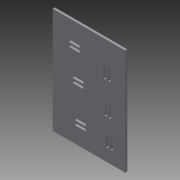
# Autodesk Inventor part: Bottom
Saved by Autodesk Inventor 2015 (Build 190159000, 159)
## iProperties
Created: 2014-09-15
Part Number: Bottom
Material: Generic
Document SubType Name: Modeling
Designer: ehagerup
Density: 1 g/cm^3
Appearance: Default
Author: ehagerup
Autodesk Inventor part; units mm, degrees
ref_plane "YZ Plane" through (0, 0, 0) normal (1, 0, 0) x (0, 1, 0)
ref_plane "XZ Plane" through (0, 0, 0) normal (0, 1, 0) x (-1, 0, 0)
ref_plane "XY Plane" through (0, 0, 0) normal (0, 0, 1) x (1, 0, 0)
sketch "Sketch1" plane through (0, 0, 0) normal (0, 1, 0) x (-1, 0, 0)
  line L0 (52.9273, -103.1635) -> (52.4273, -103.1635)
  line L1 (49.4273, -103.1635) -> (50.9273, -103.1635)
  line L2 (47.9273, -103.1635) -> (47.4273, -103.1635)
  line L3 (58.4273, -103.1635) -> (59.9273, -103.1635)
  line L4 (52.9273, -109.1635) -> (52.4273, -109.1635)
  line L5 (49.4273, -109.1635) -> (50.9273, -109.1635)
  line L6 (50.9273, -106.1635) -> (49.4273, -106.1635)
  line L7 (47.4273, -106.1635) -> (47.9273, -106.1635)
  line L8 (47.9273, -109.1635) -> (47.4273, -109.1635)
  line L9 (52.4273, -106.1635) -> (52.9273, -106.1635)
  line L10 (58.4273, -109.1635) -> (59.9273, -109.1635)
  line L11 (59.9273, -106.1635) -> (58.4273, -106.1635)
  line L12 (50.9273, -112.1635) -> (49.4273, -112.1635)
  line L13 (47.4273, -112.1635) -> (47.9273, -112.1635)
  line L14 (52.4273, -112.1635) -> (52.9273, -112.1635)
  line L15 (59.9273, -112.1635) -> (58.4273, -112.1635)
  line L16 (15.9643, -33.5509) -> (15.9643, -36.0509)
  line L17 (18.9643, -33.5509) -> (18.9643, -36.0509)
  line L18 (14.8002, -77.3245) -> (14.8002, -79.8245)
  line L19 (17.8002, -77.3245) -> (17.8002, -79.8245)
  line L20 (15.7165, -102.0792) -> (15.7165, -104.5792)
  line L21 (12.7165, -114.0792) -> (12.7165, -116.5792)
  line L22 (15.7165, -114.0792) -> (15.7165, -116.5792)
  line L23 (-7.557, 11.8403) -> (92.5214, 11.8403)
  line L24 (92.5214, 11.8403) -> (92.5214, -134.0855)
  line L25 (92.5214, -134.0855) -> (-7.557, -134.0855)
  line L26 (-7.557, -134.0855) -> (-7.557, 11.8403)
  line L27 (17.8002, -65.0745) -> (20.8002, -65.0745)
  line L28 (20.8002, -65.0745) -> (20.8002, -80.0745)
  line L29 (20.8002, -80.0745) -> (17.8002, -80.0745)
  line L30 (17.8002, -80.0745) -> (17.8002, -65.0745)
  line L31 (14.8002, -65.0745) -> (11.8002, -65.0745)
  line L32 (11.8002, -65.0745) -> (11.8002, -80.0745)
  line L33 (11.8002, -80.0745) -> (14.8002, -80.0745)
  line L34 (14.8002, -80.0745) -> (14.8002, -65.0745)
  line L35 (12.7165, -101.8292) -> (9.7165, -101.8292)
  line L36 (9.7165, -101.8292) -> (9.7165, -116.8292)
  line L37 (9.7165, -116.8292) -> (12.7165, -116.8292)
  line L38 (12.7165, -116.8292) -> (12.7165, -101.8292)
  line L39 (15.7165, -101.8292) -> (18.7165, -101.8292)
  line L40 (18.7165, -101.8292) -> (18.7165, -116.8292)
  line L41 (18.7165, -116.8292) -> (15.7165, -116.8292)
  line L42 (15.7165, -116.8292) -> (15.7165, -101.8292)
  line L43 (18.9643, -21.3009) -> (21.9643, -21.3009)
  line L44 (21.9643, -21.3009) -> (21.9643, -36.3009)
  line L45 (21.9643, -36.3009) -> (18.9643, -36.3009)
  line L46 (18.9643, -36.3009) -> (18.9643, -21.3009)
  line L47 (15.9643, -21.3009) -> (12.9643, -21.3009)
  line L48 (12.9643, -21.3009) -> (12.9643, -36.3009)
  line L49 (12.9643, -36.3009) -> (15.9643, -36.3009)
  line L50 (15.9643, -36.3009) -> (15.9643, -21.3009)
  line L51 (70.4221, -13.6009) -> (55.4221, -13.6009)
  line L52 (55.4221, -13.6009) -> (55.4221, -16.6009)
  line L53 (55.4221, -16.6009) -> (70.4221, -16.6009)
  line L54 (70.4221, -16.6009) -> (70.4221, -13.6009)
  line L55 (55.4221, -19.6009) -> (70.4221, -19.6009)
  line L56 (70.4221, -19.6009) -> (70.4221, -22.6009)
  line L57 (70.4221, -22.6009) -> (55.4221, -22.6009)
  line L58 (55.4221, -22.6009) -> (55.4221, -19.6009)
  line L59 (65.3229, -54.1341) -> (50.3229, -54.1341)
  line L60 (50.3229, -54.1341) -> (50.3229, -57.1341)
  line L61 (50.3229, -57.1341) -> (65.3229, -57.1341)
  line L62 (65.3229, -57.1341) -> (65.3229, -54.1341)
  line L63 (50.3229, -60.1341) -> (65.3229, -60.1341)
  line L64 (65.3229, -60.1341) -> (65.3229, -63.1341)
  line L65 (65.3229, -63.1341) -> (50.3229, -63.1341)
  line L66 (50.3229, -63.1341) -> (50.3229, -60.1341)
  line L67 (47.1773, -103.1635) -> (62.1773, -103.1635)
  line L68 (62.1773, -103.1635) -> (62.1773, -106.1635)
  line L69 (62.1773, -106.1635) -> (47.1773, -106.1635)
  line L70 (47.1773, -106.1635) -> (47.1773, -103.1635)
  line L71 (62.1773, -109.1635) -> (47.1773, -109.1635)
  line L72 (47.1773, -109.1635) -> (47.1773, -112.1635)
  line L73 (47.1773, -112.1635) -> (62.1773, -112.1635)
  line L74 (62.1773, -112.1635) -> (62.1773, -109.1635)
  point P0 (0, 0)
  constraints: 150 end point, 26 parallel, 13 horizontal, 13 perpendicular
extrude "Extrusion1" add sketch "Sketch1" along normal blind 3
body "Solid1"
